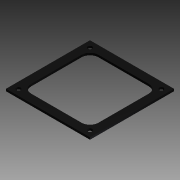
# Autodesk Inventor part: case1_space
Saved by Autodesk Inventor 2014 (Build 180170000, 170)
## iProperties
Created: 2014-02-01
Part Number: case1_space
Material: Generic
Document SubType Name: Modeling
Designer: Owner
Density: 1 g/cm^3
Appearance: Glossy - Black
Author: Owner
Autodesk Inventor part; units mm, degrees
ref_plane "YZ Plane" through (0, 0, 0) normal (1, 0, 0) x (0, 1, 0)
ref_plane "XZ Plane" through (0, 0, 0) normal (0, 1, 0) x (-1, 0, 0)
ref_plane "XY Plane" through (0, 0, 0) normal (0, 0, 1) x (1, 0, 0)
sketch "Sketch1" plane through (0, 0, 0) normal (0, 1, 0) x (-1, 0, 0)
  line L0 (-63.5, 63.5) -> (63.5, 63.5)
  line L1 (63.5, 63.5) -> (63.5, -63.5)
  line L2 (63.5, -63.5) -> (-63.5, -63.5)
  line L3 (-63.5, -63.5) -> (-63.5, 63.5)
  line L4 (-50.8, 50.8) -> (50.8, 50.8)
  line L5 (50.8, 50.8) -> (50.8, -50.8)
  line L6 (50.8, -50.8) -> (-50.8, -50.8)
  line L7 (-50.8, -50.8) -> (-50.8, 50.8)
  point P0 (0, 0)
  dimension "d0" = 127
  dimension "d1" = 127
  dimension "d2" = 63.5
  dimension "d3" = 63.5
  dimension "d4" = 50.8
  dimension "d5" = 50.8
  dimension "d6" = 101.6
  dimension "d7" = 101.6
  constraints: 16 end point, 4 parallel, 2 horizontal, 2 perpendicular
  measures "d0" distance of L0.end L1.end
  measures "d1" distance of L0.start L0.end
  measures "d2" distance from line of point (0, 0) L0
  measures "d3" distance from line of L1 point (0, 0)
  measures "d4" distance from line of point (0, 0) L4
  measures "d5" distance from line of L5 point (0, 0)
  measures "d6" distance of L4.start L4.end
  measures "d7" distance of L4.end L5.end
extrude "Extrusion1" add sketch "Sketch1" along normal blind 3.175
fillet "Fillet1" radius 12.7 4 edges at (-50.8, 1.5875, -50.8) (-50.8, 1.5875, 50.8) (50.8, 1.5875, -50.8) (50.8, 1.5875, 50.8)
sketch "Sketch2" plane through (0, 3.175, 0) normal (0, 1, 0) x (1, 0, 0)
  line L0 (63.5, 63.5) -> (-63.5, 63.5) projected
  line L1 (-63.5, 63.5) -> (-63.5, -63.5) projected
  circle A0 centre (-53.975, 53.975) radius 3.175
  circle A1 centre (53.975, 53.975) radius 3.175
  circle A2 centre (-53.975, -53.975) radius 3.175
  circle A3 centre (53.975, -53.975) radius 3.175
  point P0 (0, 0)
  dimension "d11" = 6.35
  dimension "d12" = 9.525
  dimension "d13" = 9.525
  dimension "d16" = 107.95
  dimension "d19" = 107.95
  constraints: 4 centre point, 1 horizontal, 1 vertical, 6 other
  measures "d11" diameter of A0
  measures "d12" distance from line of L1 A0.centre
  measures "d13" distance from line of L0 A0.centre
  measures "d16" distance of A0.centre A1.centre
  measures "d19" distance of A0.centre A2.centre
extrude "Extrusion2" cut sketch "Sketch2" against normal blind 3.175
body "Solid1"
